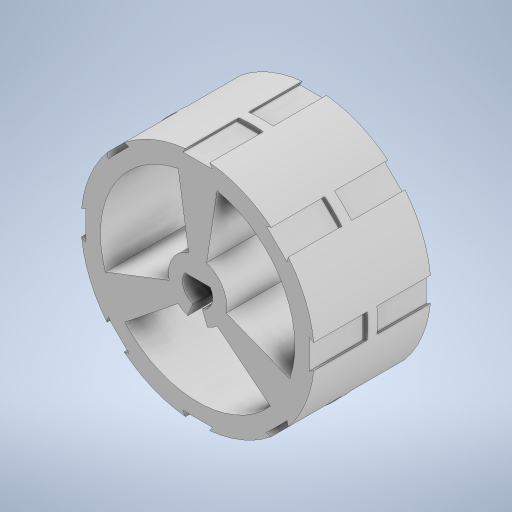
# Autodesk Inventor part: kolov2
Saved by Autodesk Inventor 2024 (Build 280153000, 153)
## iProperties
Created: 2023-10-06
Part Number: kolov2
Material: Ogólny
Document SubType Name: Modeling
Designer: Pawel
Density: 1 g/cm^3
Appearance: Domyślna
Author: Pawel
Autodesk Inventor part; units mm, degrees
ref_plane "YZ Plane" through (0, 0, 0) normal (1, 0, 0) x (0, 1, 0)
ref_plane "XZ Plane" through (0, 0, 0) normal (0, 1, 0) x (-1, 0, 0)
ref_plane "XY Plane" through (0, 0, 0) normal (0, 0, 1) x (1, 0, 0)
sketch "Szkic1" plane through (0, 0, 0) normal (0, 0, 1) x (1, 0, 0)
  circle A0 centre (0, 0) radius 12
  line L0 (-0.9273, 2.8531) -> (-2, 9.798)
  line L1 (0, 7) -> (0, 5.5022)
  line L2 (0.9273, 2.8531) -> (2, 9.798)
  line L3 (-1.3944, 1.0574) -> (1.3944, 1.0574)
  line L4 (-0.5425, -1.6638) -> (-1.0104, -2.8247)
  line L5 (0.5425, -1.6638) -> (1.0104, -2.8247)
  line L6 (-2.9345, -0.6234) -> (-9.4853, -3.1669)
  line L7 (-2.0072, -2.2296) -> (-7.4853, -6.631)
  line L8 (2.0072, -2.2296) -> (7.4853, -6.631)
  line L9 (2.9345, -0.6234) -> (9.4853, -3.1669)
  arc A1 (-2.0072, -2.2296) -> (-1.0104, -2.8247) centre (0, 0) ccw
  arc A2 (1.0104, -2.8247) -> (2.0072, -2.2296) centre (0, 0) ccw
  arc A3 (2.9345, -0.6234) -> (0.9273, 2.8531) centre (0, 0) ccw
  arc A4 (-0.9273, 2.8531) -> (-2.9345, -0.6234) centre (0, 0) ccw
  arc A5 (-2, 9.798) -> (-9.4853, -3.1669) centre (0, 0) ccw
  arc A6 (-7.4853, -6.631) -> (7.4853, -6.631) centre (0, 0) ccw
  arc A7 (9.4853, -3.1669) -> (2, 9.798) centre (0, 0) ccw
  arc A8 (0.5425, -1.6638) -> (1.3944, 1.0574) centre (0, 0) ccw
  arc A9 (-1.3944, 1.0574) -> (-0.5425, -1.6638) centre (0, 0) ccw
  point P0 (-0.7322, 1.5895)
  point P1 (0.7322, 1.5895)
  dimension "d7" = 360
  constraints: 20 end point, 18 point on circle, 10 centre point, 4 coincident, 2 symmetric about line, 1 horizontal, 1 vertical, 19 other
extrude "Wyciągnięcie proste1" add sketch "Szkic1" along normal blind 12
thicken "Pogrubienie1" operation add thickness 0.2 both sides no extend neighbours no toward (0.8822923, -0.4707019, 0) faces at (-1.544, 0.8237, 8) (-0.4648, 1.0574, 4)
thicken "Pogrubienie2" operation add thickness 0.2 both sides no extend neighbours no toward (-0.7647411, 0.6443377, 0) faces at (1.3383, -1.1276, 8)
sketch "Szkic2" plane through (0, 0, 12) normal (0, 0, 1) x (1, 0, 0)
  circle A0 centre (0, 0) radius 12 projected
  line L0 (-1.25, 11.9347) -> (-1.5, 11.5)
  line L1 (-1.5, 11.5) -> (0, 11.5)
  line L2 (-1.25, 11.9347) -> (0, 12.25)
  line L3 (0, 12) -> (0, 11.8318)
  line L4 (1.25, 11.9347) -> (1.5, 11.5)
  line L5 (1.5, 11.5) -> (0, 11.5)
  line L6 (1.25, 11.9347) -> (0, 12.25)
  line L7 (-7.0711, 9.1924) -> (-8.1317, 8.1317)
  line L8 (-9.1924, 7.0711) -> (-8.1317, 8.1317)
  line L9 (-9.323, 7.5552) -> (-9.1924, 7.0711)
  line L10 (-9.323, 7.5552) -> (-8.6621, 8.6621)
  line L11 (-7.5552, 9.323) -> (-8.6621, 8.6621)
  line L12 (-7.5552, 9.323) -> (-7.0711, 9.1924)
  line L13 (-11.5, 1.5) -> (-11.5, 0)
  line L14 (-11.5, -1.5) -> (-11.5, 0)
  line L15 (-11.9347, -1.25) -> (-11.5, -1.5)
  line L16 (-11.9347, -1.25) -> (-12.25, 0)
  line L17 (-11.9347, 1.25) -> (-12.25, 0)
  line L18 (-11.9347, 1.25) -> (-11.5, 1.5)
  line L19 (-9.1924, -7.0711) -> (-8.1317, -8.1317)
  line L20 (-7.0711, -9.1924) -> (-8.1317, -8.1317)
  line L21 (-7.5552, -9.323) -> (-7.0711, -9.1924)
  line L22 (-7.5552, -9.323) -> (-8.6621, -8.6621)
  line L23 (-9.323, -7.5552) -> (-8.6621, -8.6621)
  line L24 (-9.323, -7.5552) -> (-9.1924, -7.0711)
  line L25 (-1.5, -11.5) -> (0, -11.5)
  line L26 (1.5, -11.5) -> (0, -11.5)
  line L27 (1.25, -11.9347) -> (1.5, -11.5)
  line L28 (1.25, -11.9347) -> (0, -12.25)
  line L29 (-1.25, -11.9347) -> (0, -12.25)
  line L30 (-1.25, -11.9347) -> (-1.5, -11.5)
  line L31 (7.0711, -9.1924) -> (8.1317, -8.1317)
  line L32 (9.1924, -7.0711) -> (8.1317, -8.1317)
  line L33 (9.323, -7.5552) -> (9.1924, -7.0711)
  line L34 (9.323, -7.5552) -> (8.6621, -8.6621)
  line L35 (7.5552, -9.323) -> (8.6621, -8.6621)
  line L36 (7.5552, -9.323) -> (7.0711, -9.1924)
  line L37 (11.5, -1.5) -> (11.5, 0)
  line L38 (11.5, 1.5) -> (11.5, 0)
  line L39 (11.9347, 1.25) -> (11.5, 1.5)
  line L40 (11.9347, 1.25) -> (12.25, 0)
  line L41 (11.9347, -1.25) -> (12.25, 0)
  line L42 (11.9347, -1.25) -> (11.5, -1.5)
  line L43 (9.1924, 7.0711) -> (8.1317, 8.1317)
  line L44 (7.0711, 9.1924) -> (8.1317, 8.1317)
  line L45 (7.5552, 9.323) -> (7.0711, 9.1924)
  line L46 (7.5552, 9.323) -> (8.6621, 8.6621)
  line L47 (9.323, 7.5552) -> (8.6621, 8.6621)
  line L48 (9.323, 7.5552) -> (9.1924, 7.0711)
  dimension "d17" = 360
  constraints: 98 end point, 2 coincident, 2 symmetric about line, 1 vertical, 105 other
extrude "Wyciągnięcie proste2" cut sketch "Szkic2" against normal blind 12 contours A0 L42 L37 L38 L39 | A0 L40 L41 | L48 L43 L44 L45 A0 | A0 L46 L47 | L34 L35 A0 | A0 L36 L31 L32 L33 | L4 L5 L1 L0 A0 | A0 L2 L6 | L28 L29 A0 | A0 L30 L25 L26 L27 | L22 L23 A0 | A0 L24 L19 L20 L21 | L12 L7 L8 L9 A0 | A0 L10 L11 | L16 L17 A0 | A0 L18 L13 L14 L15
sketch "Szkic3" plane through (0, 0, 12) normal (0, 0, 1) x (1, 0, 0)
  circle A0 centre (0, 14.25) radius 0.559
  point P0 (0, 0)
  constraints: 1 centre point
extrude "Wyciągnięcie proste3" add sketch "Szkic3" against normal blind 6
sketch "Szkic4" plane through (0, 14.25, 6) normal (0, 0, -1) x (-1, 0, 0)
  arc A0 (0.4805, -15.7236) -> (1.2913, -13.3926) centre (0, -14.25) ccw projected
  circle A1 centre (0, -14.25) radius 12
  arc A2 (2.9345, -14.8734) -> (0.9273, -11.3969) centre (0, -14.25) ccw projected
  circle A3 centre (0, -14.25) radius 10.0125
  constraints: 2 centre point, 2 coincident
extrude "Wyciągnięcie proste4" add sketch "Szkic4" along normal mid plane 1
sketch "Szkic5" plane through (0, 14.25, 6) normal (0, 0, -1) x (-1, 0, 0)
  circle A0 centre (0, 0) radius 1
  point P0 (0, -14.25)
  constraints: 1 centre point
extrude "Wyciągnięcie proste5" cut sketch "Szkic5" against normal blind 12
